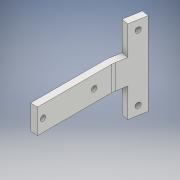
# Autodesk Inventor part: 옆면PSD받침대
Saved by Autodesk Inventor 2017 (Build 210142000, 142)
## iProperties
Part Number: 옆면PSD받침대
Material: ABS 플라스틱
Document SubType Name: Modeling
Designer: minom
Mass: 4.86164 g
Surface Area: 33.0281 cm^2
Volume: 4.58645 cm^3
Density: 1.06 g/cm^3
Appearance: 매끄러움 - 흰색
Author: minom
Autodesk Inventor part; units mm, degrees
note: some values were not read from the file. Chosen so that the rebuilt part matches the saved one: bend side of "굽힘1".
ref_plane "YZ Plane" through (0, 0, 0) normal (1, 0, 0) x (0, 1, 0)
ref_plane "XZ Plane" through (0, 0, 0) normal (0, 1, 0) x (-1, 0, 0)
ref_plane "XY Plane" through (0, 0, 0) normal (0, 0, 1) x (1, 0, 0)
sketch "스케치1" plane through (0, 0, 0) normal (1, 0, 0) x (0, 1, 0)
  line L0 (0, 0) -> (50, 0)
  line L1 (50, 0) -> (50, -14)
  line L2 (50, -14) -> (0, -14)
  line L3 (0, -14) -> (0, 0)
  circle A0 centre (32, -7) radius 1.5
  circle A1 centre (3, -7) radius 1.5
  line L4 (60, 16.5) -> (50, 16.5)
  line L5 (50, 16.5) -> (50, -30.5)
  line L6 (50, -30.5) -> (60, -30.5)
  line L7 (60, -30.5) -> (60, 16.5)
  circle A2 centre (55, 11.5) radius 1.5
  circle A3 centre (55, -25.5) radius 1.5
  point P0 (50, -7)
  dimension "d0" = 50
  dimension "d1" = 14
  dimension "d2" = 3
  dimension "d3" = 3
  dimension "d4" = 29
  dimension "d5" = 7
  dimension "d6" = 7
  dimension "d10" = 3
  dimension "d11" = 10
  dimension "d12" = 47
  dimension "d13" = 3
  dimension "d14" = 3
  dimension "d15" = 37
  dimension "d16" = 5
  dimension "d17" = 5
  dimension "d18" = 5
  constraints: 16 end point, 4 centre point, 4 parallel, 2 horizontal, 2 midpoint, 2 perpendicular
  measures "d0" distance of L1.end L2.end
  measures "d1" distance of L0.end L1.end
  measures "d2" diameter of A0
  measures "d3" diameter of A1
  measures "d4" distance of A1.centre A0.centre
  measures "d5" distance from line of L0 A0.centre
  measures "d6" distance from line of L2 A1.centre
  measures "d10" distance from line of L3 A1.centre
  measures "d11" distance of L6.end L5.end
  measures "d12" distance of L5.end L4.end
  measures "d13" diameter of A2
  measures "d14" diameter of A3
  measures "d15" distance of A3.centre A2.centre
  measures "d16" distance from line of L4 A2.centre
  measures "d17" distance from line of L7 A2.centre
  measures "d18" distance from line of L5 A3.centre
extrude "돌출2" add sketch "스케치1" along normal blind 4
sketch "스케치2" plane through (4, 0, 0) normal (1, 0, 0) x (0, 0, -1)
  circle A0 centre (7, 3) radius 1.5 projected
  circle A1 centre (7, 32) radius 1.5 projected
  circle A2 centre (25.5, 55) radius 1.5 projected
  circle A3 centre (-11.5, 55) radius 1.5 projected
  line L0 (-16.5, 50) -> (0, 50) projected
  line L1 (0, 50) -> (0, 0) projected
  line L2 (0, 0) -> (14, 0) projected
  line L3 (14, 0) -> (14, 50) projected
  line L4 (14, 50) -> (30.5, 50) projected
  line L5 (30.5, 50) -> (30.5, 60) projected
  line L6 (30.5, 60) -> (-16.5, 60) projected
  line L7 (-16.5, 60) -> (-16.5, 50) projected
  line L8 (0, 50) -> (0, 0) projected
  line L9 (0, 42) -> (14, 42)
  line L10 (14, 0) -> (14, 50) projected
  dimension "d21" = 10
  constraints: 2 end point, 2 point on line, 1 horizontal
  measures "d21" distance from line of L9 A1.centre
bend part "굽힘1" radius 10 angle 10 line through (4, 42, 0) along (0, 0, -1) centre toward (1, 0, 0) moving side (0, 1, 0) both sides no
